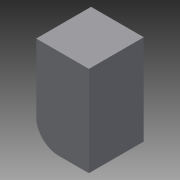
# Autodesk Inventor part: test
Saved by Autodesk Inventor 2015 (Build 190159000, 159)
## iProperties
Created: 2014-07-13
Part Number: test
Material: Generic
Document SubType Name: Modeling
Designer: shohei
Density: 1 g/cm^3
Appearance: Default
Author: shohei
Autodesk Inventor part; units mm, degrees
ref_plane "YZ Plane" through (0, 0, 0) normal (1, 0, 0) x (0, 1, 0)
ref_plane "XZ Plane" through (0, 0, 0) normal (0, 1, 0) x (-1, 0, 0)
ref_plane "XY Plane" through (0, 0, 0) normal (0, 0, 1) x (1, 0, 0)
sketch "Sketch1" plane through (0, 0, 0) normal (0, 1, 0) x (-1, 0, 0)
  line L0 (0, 0) -> (0, -16.4523)
  line L1 (0, -16.4523) -> (5.537, -16.4523)
  arc A0 (5.537, -16.4523) -> (9.5985, -12.6447) centre (5.537, -12.3824) ccw
  line L2 (9.5985, -12.6447) -> (9.5985, 0)
  line L3 (9.5985, 0) -> (0, 0)
  constraints: 8 end point, 3 perpendicular, 2 point on circle, 1 centre point, 1 tangent, 1 vertical
extrude "Extrusion1" add sketch "Sketch1" along normal blind 10
body "Solid1"
